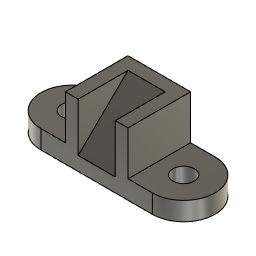
A2 object v1 (Autodesk Fusion 360 design; units mm, degrees)
Autodesk Fusion 360 part; units mm, degrees
sketch "Sketch1" plane through (0, 0, 0) normal (0, 0, 1) x (1, 0, 0)
  line L0 (57, -32) -> (-57, -32)
  line L1 (-57, 32) -> (57, 32)
  circle A0 centre (57, 0) radius 11
  circle A1 centre (-57, 0) radius 11
  arc A2 (57, -32) -> (57, 32) centre (57, 0) ccw
  arc A3 (-57, 32) -> (-57, -32) centre (-57, 0) ccw
  dimension "d1" = 114
  dimension "d2" = 64
  dimension "d3" = 32
  dimension "d4" = 22
  dimension "d5" = 32
  dimension "d6" = 22
  constraint horizontal L0
  constraint parallel L0 L1
  constraint concentric A0 A2
  constraint concentric A1 A3
  measures "d1" distance of L1.start L1.end
  measures "d2" distance of L0.end L1.start
  measures "d3" radius of A2
  measures "d4" diameter of A0
  measures "d5" radius of A3
  measures "d6" diameter of A1
extrude "Extrude1" add sketch "Sketch1" along normal blind 19
sketch "Sketch2" plane through (0, 0, 0) normal (0, 1, 0) x (1, 0, 0)
  line L0 (-32, -0.1347) -> (32, -0.1347)
  line L1 (32, -0.1347) -> (32, -64.1347)
  line L2 (32, -64.1347) -> (-32, -64.1347)
  line L3 (-32, -64.1347) -> (-32, -0.1347)
  line L4 (-57, 0) -> (-57, -19)
  dimension "d9" = 64
  dimension "d10" = 64
  dimension "d11" = 25
  constraint horizontal L0
  constraint vertical L1
  constraint horizontal L2
  constraint vertical L3
  measures "d9" distance of L0.start L0.end
  measures "d10" distance of L0.start L2.end
  measures "d11" distance of L3 L4
extrude "Extrude2" add sketch "Sketch2" along normal mid plane 64
sketch "Sketch3" plane through (0, 0, 64.1347) normal (0, 0, 1) x (-1, 0, 0)
  line L0 (-32, 32) -> (-32, -32)
  line L1 (-32, -32) -> (32, -32)
  line L2 (32, -32) -> (32, 32)
  line L3 (32, 32) -> (-32, 32)
  line L4 (-19, 32) -> (-19, -19)
  line L5 (-19, -19) -> (19, -19)
  line L6 (19, -19) -> (19, 32)
  line L7 (-19, 32) -> (19, 32)
  dimension "d14" = 51
  dimension "d15" = 38
  dimension "d16" = 51
  dimension "d17" = 13
  dimension "d22" = 13
  dimension "d23" = 13
  constraint coincident L3 L4.start
  constraint perpendicular L3 L4
  constraint perpendicular L4 L5
  constraint perpendicular L3 L6
  measures "d14" distance of L4.start L4.end
  measures "d15" distance of L4.end L5.end
  measures "d16" distance of L5.end L6.end
  measures "d17" distance of L1 L5.end
  measures "d22" distance of L0 L4
  measures "d23" distance of L2 L6
extrude "Extrude3" cut sketch "Sketch3" against normal blind 50 contours L3 L4 L5 L6 L7
draft "Draft1" angle 45.6 neutral plane through (32, 0, 64.1347) pull (0, 0, 1) 1 faces at (6.3333, 19, 47.468)
named bodies: "A2"
